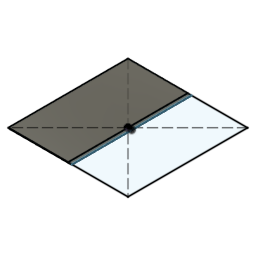
2024_10_12_PediluveShort v2 (Autodesk Fusion 360 design; units mm, degrees)
Autodesk Fusion 360 part; units mm, degrees
sketch "Sketch1" plane through (0, 0, 0) normal (0, 0, 1) x (1, 0, 0)
sketch "32MPediluveSplitter" plane through (0, 0, 0) normal (0, 0, 1) x (1, 0, 0)
  line L0 (32767.5, 32767.5) -> (-32767.5, 32767.5)
  line L1 (-32767.5, 32767.5) -> (-32767.5, -32767.5)
  line L2 (-32767.5, -32767.5) -> (32767.5, -32767.5)
  line L3 (32767.5, -32767.5) -> (32767.5, 32767.5)
  line L4 (32767.5, 32767.5) -> (-32767.5, -32767.5) construction
  line L5 (-32767.5, 32767.5) -> (32767.5, -32767.5) construction
  line L6 (0, 0) -> (0, 32767.5)
  line L7 (0, 0) -> (0, -32767.5)
  line L8 (0, 0) -> (2000, 0)
  line L9 (2000, 32767.5) -> (2000, -32767.5)
  dimension "d5" = 65535
  dimension "d6" = 65535
  dimension "d7" = 2000
  constraint horizontal L0
  constraint perpendicular L0 L1
  constraint parallel L0 L2
  constraint parallel L1 L3
  constraint coincident L4 L6.start
  constraint coincident L5 L6.start
  constraint coincident L6.start L7.start
  constraint midpoint L0 L6.end
  constraint midpoint L2 L7.end
  constraint horizontal L8
  constraint coincident L0 L9.start
  constraint coincident L2 L9.end
  constraint perpendicular L2 L9
  measures "d5" distance of L1.end L2.end
  measures "d6" distance of L0.end L1.end
  measures "d7" distance of L6.start L8.end
extrude "Extrude1" add sketch "32MPediluveSplitter" along normal blind 0.3 contours L0 L2 L3 L9 makes body 1
extrude "Extrude2" add sketch "32MPediluveSplitter" along normal blind 100 separate body contours L0 L1 L2 L6 L7 makes body 2
extrude "Extrude3" add sketch "32MPediluveSplitter" 1 faces at (-21845, 0, 0) along normal blind 0.3 contours L0 L6 L8 L9 | L0 L1 L2 L6 L7 | L2 L7 L8 L9 on bodies 2 bodies 1 2
extrude "Extrude4" cut sketch "32MPediluveSplitter" along normal blind 6000 contours L0 L2 L3 L9 bodies 1
extrude "Extrude5" add sketch "32MPediluveSplitter" against normal blind 300 contours L0 L6 L8 L9 | L0 L1 L2 L6 L7 | L2 L7 L8 L9 bodies 1
equation "short = 1 mm + ( 32767 * 2 ) * 1 mm"
equation "halfshort = short / 2"
equation "d5 = short"
equation "d6 = short"
named bodies: "PediluveGround"
